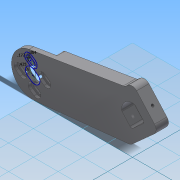
# Autodesk Inventor part: MountSketch
Saved by Autodesk Inventor 2014 SP2 (Build 180246200, 246)
## iProperties
Created: 2014-05-16
Part Number: MountSketch
Material: Generic
Document SubType Name: Modeling
Designer: dliu
Density: 1 g/cm^3
Appearance: Default
Author: dliu
Autodesk Inventor part; units mm, degrees
note: some values were not read from the file. Chosen so that the rebuilt part matches the saved one: direction of "Hole3"; direction of "Hole4".
ref_plane "YZ Plane" through (0, 0, 0) normal (1, 0, 0) x (0, 1, 0)
sketch "the Axle" plane through (0, 0, 0) normal (0, 0, 1) x (1, 0, 0)
  line L0 (-30.4731, 63.7704) -> (-43.9693, 51.6183)
  line L1 (-43.9693, 51.6183) -> (-54.1341, 62.9075)
  line L2 (-40.6378, 75.0595) -> (-30.4731, 63.7704)
  line L3 (-30.4731, 63.7704) -> (-12.3121, 63.7704) construction
  arc A0 (-40.6378, 75.0595) -> (-54.1341, 62.9075) centre (-42.9621, 64.0703) ccw
  line L4 (-54.1341, 62.9075) -> (-40.6378, 75.0595) construction
  point P0 (-12.6671, 65.6222)
  dimension "d84" = 18.161
  dimension "d85" = 138
  dimension "d231" = 19.812
  measures "d84" distance of L2.end L1.start
  measures "d85" angle of L0 L3
sketch "Motor Mount Pattern" plane through (0, 0, 0) normal (0, 0, 1) x (1, 0, 0)
  line L0 (-116.3697, 51.2894) -> (-116.3697, 68.9671) construction
  line L1 (-116.3697, 68.9671) -> (-134.0474, 68.9671) construction
  line L2 (-134.0474, 68.9671) -> (-134.0474, 51.2894) construction
  line L3 (-134.0474, 51.2894) -> (-116.3697, 68.9671) construction
  line L4 (-116.3697, 51.2894) -> (-134.0474, 68.9671) construction
  line L5 (-134.0474, 51.2894) -> (-134.0474, 68.9671) construction
  line L6 (-134.0474, 51.2894) -> (-116.3697, 68.9671) construction
  line L7 (-134.0474, 51.2894) -> (-125.2086, 60.1282) construction
  line L8 (-116.3697, 51.2894) -> (-134.0474, 51.2894) construction
  circle A0 centre (-125.2086, 60.1282) radius 6.2
  circle A1 centre (-116.3697, 68.9671) radius 2.25
  circle A2 centre (-134.0474, 68.9671) radius 2.25
  circle A3 centre (-116.3697, 51.2894) radius 2.25
  circle A4 centre (-134.0474, 51.2894) radius 2.25
  circle A5 centre (-116.3697, 68.9671) radius 4.5 construction
  circle A6 centre (-134.0474, 68.9671) radius 4.5 construction
  circle A7 centre (-134.0474, 51.2894) radius 4.5 construction
  circle A8 centre (-116.3697, 51.2894) radius 4.5 construction
  point P0 (-121.7102, 57.8126)
  dimension "d189" = 25
  dimension "d192" = 12.4
  dimension "d193" = 4.5
  dimension "d195" = 9
  measures "d189" distance of L0.start L1.end
  measures "d192" diameter of A0
  measures "d193" diameter of A1
  measures "d195" diameter of A5
sketch "Motor Body Extent" plane through (0, 0, 0) normal (0, 0, 1) x (1, 0, 0)
  circle A0 centre (-176.4641, 62.233) radius 24.5 construction
  dimension "MotorDia" = 49
  measures "MotorDia" diameter of A0
sketch "Block7" plane through (0, 0, 0) normal (0, 0, 1) x (1, 0, 0)
  line L0 (-114.6206, 39.8537) -> (-104.0422, 54.0169) construction
  line L1 (-104.0422, 54.0169) -> (-118.2054, 64.5953) construction
  line L2 (-118.2054, 64.5953) -> (-128.7838, 50.432) construction
  line L3 (-128.7838, 50.432) -> (-104.0422, 54.0169) construction
  line L4 (-114.6206, 39.8537) -> (-118.2054, 64.5953) construction
  line L5 (-128.7838, 50.432) -> (-118.2054, 64.5953) construction
  line L6 (-128.7838, 50.432) -> (-104.0422, 54.0169) construction
  line L7 (-128.7838, 50.432) -> (-116.413, 52.2245) construction
  line L8 (-114.6206, 39.8537) -> (-128.7838, 50.432) construction
  circle A0 centre (-116.413, 52.2245) radius 6.2
  circle A1 centre (-104.0422, 54.0169) radius 2.25
  circle A2 centre (-118.2054, 64.5953) radius 2.25
  circle A3 centre (-114.6206, 39.8537) radius 2.25
  circle A4 centre (-128.7838, 50.432) radius 2.25
  circle A5 centre (-104.0422, 54.0169) radius 4.5 construction
  circle A6 centre (-118.2054, 64.5953) radius 4.5 construction
  circle A7 centre (-128.7838, 50.432) radius 4.5 construction
  circle A8 centre (-114.6206, 39.8537) radius 4.5 construction
  line L9 (-107.5171, 56.2696) -> (-121.6653, 66.8681) construction
  line L10 (-121.6653, 66.8681) -> (-132.2638, 52.7199) construction
  line L11 (-132.2638, 52.7199) -> (-118.1156, 42.1214) construction
  line L12 (-118.1156, 42.1214) -> (-121.6653, 66.8681) construction
  line L13 (-107.5171, 56.2696) -> (-132.2638, 52.7199) construction
  line L14 (-118.1156, 42.1214) -> (-132.2638, 52.7199) construction
  line L15 (-118.1156, 42.1214) -> (-121.6653, 66.8681) construction
  line L16 (-118.1156, 42.1214) -> (-119.8904, 54.4948) construction
  line L17 (-107.5171, 56.2696) -> (-118.1156, 42.1214) construction
  circle A9 centre (-119.8904, 54.4948) radius 6.2
  circle A10 centre (-121.6653, 66.8681) radius 2.25
  circle A11 centre (-132.2638, 52.7199) radius 2.25
  circle A12 centre (-107.5171, 56.2696) radius 2.25
  circle A13 centre (-118.1156, 42.1214) radius 2.25
  circle A14 centre (-121.6653, 66.8681) radius 4.5 construction
  circle A15 centre (-132.2638, 52.7199) radius 4.5 construction
  circle A16 centre (-118.1156, 42.1214) radius 4.5 construction
  circle A17 centre (-107.5171, 56.2696) radius 4.5 construction
  line L18 (-105.811, 55.3186) -> (-120.0113, 65.8472) construction
  line L19 (-120.0113, 65.8472) -> (-130.5399, 51.6469) construction
  line L20 (-130.5399, 51.6469) -> (-116.3396, 41.1183) construction
  line L21 (-116.3396, 41.1183) -> (-120.0113, 65.8472) construction
  line L22 (-105.811, 55.3186) -> (-130.5399, 51.6469) construction
  line L23 (-116.3396, 41.1183) -> (-130.5399, 51.6469) construction
  line L24 (-116.3396, 41.1183) -> (-120.0113, 65.8472) construction
  line L25 (-116.3396, 41.1183) -> (-118.1755, 53.4828) construction
  line L26 (-105.811, 55.3186) -> (-116.3396, 41.1183) construction
  circle A18 centre (-118.1755, 53.4828) radius 6.2
  circle A19 centre (-120.0113, 65.8472) radius 2.25
  circle A20 centre (-130.5399, 51.6469) radius 2.25
  circle A21 centre (-105.811, 55.3186) radius 2.25
  circle A22 centre (-116.3396, 41.1183) radius 2.25
  circle A23 centre (-120.0113, 65.8472) radius 4.5 construction
  circle A24 centre (-130.5399, 51.6469) radius 4.5 construction
  circle A25 centre (-116.3396, 41.1183) radius 4.5 construction
  circle A26 centre (-105.811, 55.3186) radius 4.5 construction
  point P0 (-115.0557, 53.032)
sketch "MotorMountPattern" plane through (0, 0, 0) normal (0, 0, 1) x (1, 0, 0)
  line L0 (-95.4079, 16.8905) -> (-77.7418, 16.8905) construction
  line L1 (-77.7418, 16.8905) -> (-77.7418, 34.5797) construction
  line L2 (-77.7418, 34.5797) -> (-95.4079, 34.5797) construction
  line L3 (-95.4079, 34.5797) -> (-95.4079, 16.8905)
  line L4 (-95.4079, 16.8905) -> (-77.7418, 34.5797) construction
  line L5 (-77.7418, 16.8905) -> (-95.4079, 34.5797) construction
  line L6 (-86.5749, 25.7351) -> (-91.6549, 25.7351)
  line L7 (-95.4079, 34.5797) -> (-100.4879, 34.5797)
  line L8 (-95.4079, 16.8905) -> (-100.4879, 16.8905)
  line L9 (-77.7418, 34.5797) -> (-82.8218, 34.5797)
  line L10 (-77.7418, 16.8905) -> (-82.8218, 16.8905)
  point P0 (-89.1149, 25.7351)
  dimension "d197" = 25
  dimension "Adjustability" = 5.08
  measures "d197" distance of L8.start L9.start
  measures "Adjustability" distance of L6.start L6.end
sketch "Base Sketch" plane through (0, 0, 0) normal (0, 0, 1) x (1, 0, 0)
  line L0 (26.8378, -1.0519) -> (-1.7592, -26.8007)
  line L1 (-1.7592, -26.8007) -> (-28.6127, 3.0232)
  line L2 (-28.6127, 3.0232) -> (-0.0158, 28.772)
  line L3 (-0.0158, 28.772) -> (26.8378, -1.0519)
  line L4 (-7.5661, 21.9736) -> (19.2874, -7.8503)
  circle A0 centre (0, 0) radius 41.5 construction
  line L5 (-7.5661, 21.9736) -> (-105.9285, 5.8665)
  line L6 (-100.2333, -36.9167) -> (-1.7592, -26.8007)
  circle A1 centre (-102.4396, -15.4397) radius 21.59
  line L7 (-148.6125, -66.8274) -> (67.2297, -66.8274) construction
  circle A2 centre (-100.3809, -16.9274) radius 24.5 construction
  line L8 (12.489, -0.2999) -> (-1.0072, -12.452)
  line L9 (-1.0072, -12.452) -> (-11.172, -1.1629)
  line L10 (2.3243, 10.9892) -> (12.489, -0.2999)
  line L11 (12.489, -0.2999) -> (30.65, -0.2999) construction
  arc A3 (2.3243, 10.9892) -> (-11.172, -1.1629) centre (0, 0) ccw
  line L12 (-11.172, -1.1629) -> (2.3243, 10.9892) construction
  line L13 (-112.7206, -18.9225) -> (-98.4019, -29.2698) construction
  line L14 (-98.4019, -29.2698) -> (-88.0411, -14.9323) construction
  line L15 (-88.0411, -14.9323) -> (-102.3599, -4.585) construction
  line L16 (-102.3599, -4.585) -> (-112.7206, -18.9225)
  line L17 (-112.7206, -18.9225) -> (-88.0411, -14.9323) construction
  line L18 (-98.4019, -29.2698) -> (-102.3599, -4.585) construction
  line L19 (-100.3809, -16.9274) -> (-104.4983, -13.952)
  line L20 (-102.3599, -4.585) -> (-106.4773, -1.6096)
  line L21 (-112.7206, -18.9225) -> (-116.8381, -15.9471)
  line L22 (-88.0411, -14.9323) -> (-92.1586, -11.9569)
  line L23 (-98.4019, -29.2698) -> (-102.5193, -26.2943)
  dimension "AxleMargin" = 10.16
  dimension "d97" = 10.16
  dimension "d98" = 10.16
  dimension "d99" = 10.16
  dimension "WheelDia" = 83
  dimension "d157" = 43.18
  dimension "NomCtrDist" = 101.7981
  dimension "d209" = 105.4256
  dimension "AxleBoardClearance" = 66.8274
  dimension "d233" = 49
  dimension "BoardClearance" = 25.4
  constraints: 16 end point, 4 point on line, 3 centre point, 2 coincident, 2 parallel, 2 perpendicular, 2 point on circle, 2 tangent, 1 horizontal, 5 other
  measures "WheelDia" diameter of A0
  measures "d157" diameter of A1
  measures "AxleBoardClearance" distance from line of point (0, 0) L7
  measures "d233" diameter of A2
  measures "BoardClearance" distance edge to line of A2 L7
extrude "Base" add sketch "Base Sketch" against normal blind 12.7 contours L0 L4 L2 L3 | L0 L1 L2 L4 A3 L9 L8 | L6 A1 L5 L2 L1 | A1
sketch "Motor Hole Sketch" plane through (0, 0, 0) normal (0, 0, 1) x (1, 0, 0)
  line L0 (-102.3599, -4.585) -> (-106.4773, -1.6096) construction
  line L1 (-101.042, -2.7614) -> (-105.1594, 0.214)
  line L2 (-107.7952, -3.4333) -> (-103.6777, -6.4087)
  arc A0 (-103.6777, -6.4087) -> (-101.042, -2.7614) centre (-102.3599, -4.585) ccw
  arc A1 (-105.1594, 0.214) -> (-107.7952, -3.4333) centre (-106.4773, -1.6096) ccw
  line L3 (-100.3809, -16.9274) -> (-104.4983, -13.952) construction
  line L4 (-97.218, -12.5506) -> (-101.3355, -9.5752)
  line L5 (-107.6612, -18.3288) -> (-103.5437, -21.3042)
  arc A2 (-103.5437, -21.3042) -> (-97.218, -12.5506) centre (-100.3809, -16.9274) ccw
  arc A3 (-101.3355, -9.5752) -> (-107.6612, -18.3288) centre (-104.4983, -13.952) ccw
  line L6 (-102.3599, -4.585) -> (-106.4773, -1.6096) construction
  line L7 (-99.7242, -0.9377) -> (-103.8416, 2.0377)
  line L8 (-109.113, -5.257) -> (-104.9956, -8.2324)
  arc A4 (-104.9956, -8.2324) -> (-99.7242, -0.9377) centre (-102.3599, -4.585) ccw
  arc A5 (-103.8416, 2.0377) -> (-109.113, -5.257) centre (-106.4773, -1.6096) ccw
  point P0 (-104.4186, -3.0973)
  point P1 (-102.4396, -15.4397)
  point P2 (-104.4186, -3.0973)
  dimension "M4ClearanceDia" = 4.5
  dimension "d211" = 10.8
  dimension "d218" = 9
  constraints: 24 end point, 12 point on circle, 12 tangent, 6 centre point, 5 equal length, 3 midpoint
  measures "M4ClearanceDia" diameter of A1
  measures "d211" diameter of A3
  measures "d218" diameter of A5
extrude "Motor Hole" cut sketch "Motor Hole Sketch" against normal through all contours A0 L2 A1 L1
extrude "Motor Cbore" cut sketch "Motor Hole Sketch" against normal blind 3 contours A0 L2 A1 L1 | A4 A3 | A3 A4 L8 A5 L7
pattern_linear "Rectangular Pattern1" count 2 spacing 17.6661 along (0.810519, -0.5857123, 0) count 2 spacing 17.6661 along (-0.5857123, -0.810519, 0) of "Motor Hole", "Motor Cbore"
extrude "Motor Axle" cut sketch "Motor Hole Sketch" against normal through all contours A2 L5 A3 A4 L4 | A4 A3
ref_plane "Back Plane" through (0, 0, -12.7) normal (0, 0, -1) x (-1, 0, 0)
sketch "Sketch12" plane through (0, 0, -12.7) normal (0, 0, -1) x (-1, 0, 0)
  line L0 (7.5661, 21.9736) -> (105.9285, 5.8665) projected
  line L1 (100.2333, -36.9167) -> (1.7592, -26.8007) projected
  line L2 (16.1, -21.8905) -> (20.7942, 13.3729)
  line L3 (75.7186, -28.0149) -> (16.1, -21.8905)
  line L4 (20.7942, 13.3729) -> (82.4161, 3.2822)
  line L5 (100.3809, -16.9274) -> (104.4983, -13.952) construction
  line L6 (114.7308, -36.7851) -> (118.8483, -33.8097) construction
  line L7 (90.1484, 5.9057) -> (86.0309, 2.9303) construction
  arc A0 (86.0309, 2.9303) -> (114.7308, -36.7851) centre (100.3809, -16.9274) ccw construction
  arc A1 (118.8483, -33.8097) -> (90.1484, 5.9057) centre (104.4983, -13.952) ccw construction
  line L8 (116.2185, -38.8438) -> (120.336, -35.8684)
  arc A2 (120.336, -35.8684) -> (88.6607, 7.9645) centre (104.4983, -13.952) ccw
  line L9 (88.6607, 7.9645) -> (84.5432, 4.989)
  arc A3 (84.5432, 4.989) -> (82.4161, 3.2822) centre (100.3809, -16.9274) ccw
  arc A4 (75.7186, -28.0149) -> (116.2185, -38.8438) centre (100.3809, -16.9274) ccw
  arc A5 (82.4161, 3.2822) -> (75.7186, -28.0149) centre (100.3809, -16.9274) ccw
  arc A6 (74.798, 4.5297) -> (68.6388, -27.2876) centre (100.3809, -16.9274) ccw
  point P0 (0, 0)
  point P1 (11.172, -1.1629)
  point P2 (102.4396, -15.4397)
  dimension "d178" = 7.62
  dimension "d183" = 6.35
  dimension "d186" = 88.283
  dimension "d187" = 88.283
  dimension "d226" = 6.35
  dimension "d228" = 49
  dimension "d229" = 2.54
  dimension "d251" = 6.35
  dimension "d252" = 2.54
  constraints: 18 end point, 15 point on circle, 7 centre point, 4 parallel, 4 tangent, 2 point on line, 1 midpoint, 2 other
  measures "d178" distance from line of L2 point (11.172, -1.163)
  measures "d183" distance between parallel lines of L0 L4
  measures "d186" angle of L4 L2
  measures "d187" angle of L3 L2
  measures "d226" distance between parallel lines of L1 L3
  measures "d228" diameter of A1
  measures "d229" radial gap between concentric circles of A3 A0
  measures "d251" radial gap between concentric circles of A6 A5
  measures "d252" radial gap between concentric circles of A2 A1
extrude "Pocket" cut sketch "Sketch12" against normal blind 7.9375 contours L2 L4 A6 L3 | A5 A3 L9 A2 L8 A4
ref_plane "Midplane" through (0, 0, -6.35) normal (0, 0, 1) x (1, 0, 0)
sketch "Sketch15" plane through (26.8378, -1.0519, 0) normal (0.7431448, 0.6691306, 0) x (0, 0, -1)
  line L0 (0, 18.7397) -> (6.35, 18.7397) construction
  dimension "d235" = 6.35
  constraints: 2 end point, 1 horizontal
  measures "d235" distance of L0.start L0.end
sketch "Sketch16" plane through (-1.7592, -26.8007, -12.7) normal (0.6691306, -0.7431448, 0) x (0.7431448, 0.6691306, 0)
  line L0 (19.2405, 12.7) -> (19.2405, 6.35) construction
  dimension "d236" = 6.35
  constraints: 2 end point, 1 vertical
  measures "d236" distance of L0.start L0.end
hole "Hole3" at (14.2985, 12.8744, -6.35) direction (-0.7431448, -0.6691306, 0) diameter 2.6416 end up to surface thread size "6-32 UNC" class "2B" standard "ANSI Unified Screw Threads"
hole "Hole4" at (12.5393, -13.9263, -6.35) direction (-0.6691306, 0.7431448, 0) diameter 2.6416 end up to surface thread size "6-32 UNC" class "2B" standard "ANSI Unified Screw Threads"
fillet "Fillet1" radius 6.35 4 edges at (-1.7592, -26.8007, -6.35) (-7.5661, 21.9736, -6.35) (-0.0158, 28.772, -6.35) (26.8378, -1.0519, -6.35)
fillet "Fillet2" radius 3.175 2 edges at (-89.5115, 8.5549, -8.7312) (-80.1357, -34.8521, -8.7312)
fillet "Fillet3" radius 3.175 2 edges at (-20.7942, 13.3729, -8.7312) (-16.1, -21.8905, -8.7312)
fillet "Fillet4" radius 2.286 4 edges at (12.489, -0.2999, -6.35) (-1.0072, -12.452, -6.35) (-11.172, -1.1629, -6.35) (2.3243, 10.9892, -6.35)
body "Solid5"
body "Solid4"
